Autodesk Inventor part; units mm, degrees
(part 2 of 2)
sketch "Эскиз23" plane through (0, -2, 0) normal (0, -1, 0) x (1, 0, 0)
  line L0 (-21, -26.125) -> (-21, -6.125) projected
  line L1 (-21, -16.125) -> (-28.5, -16.125) construction
  line L2 (-28.5, -13.725) -> (-33, -13.725)
  line L3 (-33, -13.725) -> (-33, -18.525)
  line L4 (-33, -18.525) -> (-28.5, -18.525)
  line L5 (-28.5, -18.525) -> (-28.5, -13.725)
  line L6 (-21, -16.125) -> (-28.5, -18.525) construction
  line L7 (-28.5, -13.725) -> (-21, -16.125) construction
  point P0 (0, 0)
  dimension "d124" = 7.5
  dimension "d125" = 4.8
  dimension "d130" = 4.5
  constraints: 14 end point, 2 horizontal, 2 midpoint, 2 parallel, 1 equal length, 1 perpendicular
  measures "d124" distance of L1.start L1.end
  measures "d125" distance between parallel lines of L2 L4
  measures "d130" distance between parallel lines of L3 L5
sketch "Эскиз25" plane through (-56.2, -2, -32.25) normal (-1, 0, 0) x (0, 0, 1)
  line L0 (2.125, 0) -> (30.125, 0) construction
  line L1 (30.125, 0) -> (30.125, 47.7) construction
  line L2 (30.125, 47.7) -> (2.125, 47.7) construction
  line L3 (2.125, 47.7) -> (2.125, 0) construction
  line L4 (26.125, 43.7) -> (26.125, 4) construction
  line L5 (26.125, 4) -> (6.125, 4) construction
  line L6 (6.125, 4) -> (6.125, 43.7) construction
  line L7 (6.125, 43.7) -> (26.125, 43.7) construction
  line L8 (30.125, 47.7) -> (31.625, 49.2) construction
  line L9 (30.125, 47.7) -> (26.125, 43.7) construction
  line L10 (26.125, 4) -> (26.125, 43.7) construction
  line L11 (26.125, 4) -> (6.125, 43.7) construction
  line L12 (26.125, 43.7) -> (6.125, 4) construction
  line L13 (16.125, 23.85) -> (26.125, 23.85) construction
  line L14 (16.125, 23.85) -> (16.125, 43.7) construction
  line L15 (6.125, 43.7) -> (26.125, 43.7) construction
  circle A0 centre (27.7819, 45.3569) radius 2.3431 construction
  circle A1 centre (27.7819, 45.3569) radius 1.05
  circle A2 centre (4.4681, 45.3569) radius 1.05
  circle A3 centre (27.7819, 2.3431) radius 1.05
  circle A4 centre (4.4681, 2.3431) radius 1.05
  point P0 (32.25, 2)
  dimension "d131" = 2.1
  constraints: 10 end point, 4 centre point, 3 midpoint, 3 symmetric about line, 1 coincident, 1 collinear, 1 horizontal, 1 point on line, 6 other
  measures "d131" diameter of A1
sketch "Эскиз26" plane through (-46.2, -2, -32.25) normal (-1, 0, 0) x (0, 0, 1)
  circle A0 centre (21.0926, -11.2426) radius 1.05
  line L0 (2.125, 47.7) -> (30.125, 47.7) projected
  circle A1 centre (4.4681, 45.3569) radius 1.05 projected
  line L1 (6.1624, 47.0511) -> (6.7825, 44.7367)
  line L2 (6.7825, 44.7367) -> (5.0883, 43.0425)
  line L3 (5.0883, 43.0425) -> (2.7739, 43.6626)
  line L4 (2.7739, 43.6626) -> (2.1538, 45.977)
  line L5 (2.1538, 45.977) -> (3.848, 47.6712)
  line L6 (3.848, 47.6712) -> (6.1624, 47.0511)
  line L7 (26.125, 43.7) -> (6.125, 43.7) projected
  line L8 (6.7825, 44.7367) -> (9.7458, 47.7)
  line L9 (9.7458, 47.7) -> (6.8113, 50.6345)
  line L10 (6.8113, 50.6345) -> (3.848, 47.6712)
  circle A2 centre (4.4681, 2.3431) radius 1.05 projected
  circle A3 centre (4.4681, 45.3569) radius 1.05 projected
  circle A4 centre (27.7819, 45.3569) radius 1.05 projected
  circle A5 centre (27.7819, 2.3431) radius 1.05 projected
  line L11 (2.125, 0) -> (30.125, 0) projected
  line L12 (30.125, 0) -> (30.125, 47.7) projected
  line L13 (30.125, 47.7) -> (2.125, 47.7) projected
  line L14 (2.125, 47.7) -> (2.125, 0) projected
  line L15 (26.125, 43.7) -> (26.125, 4) projected
  line L16 (26.125, 4) -> (6.125, 4) projected
  line L17 (6.125, 4) -> (6.125, 43.7) projected
  line L18 (6.125, 43.7) -> (26.125, 43.7) projected
  line L19 (30.125, 47.7) -> (30.125, 0) projected
  line L20 (0.625, 0) -> (2.125, 0) projected
  line L21 (30.125, 47.7) -> (2.125, 0) construction
  line L22 (16.125, 23.85) -> (23.6976, 23.85) construction
  line L23 (16.125, 23.85) -> (16.125, 29.0933) construction
  circle A6 centre (27.7819, 45.3569) radius 1.05
  line L24 (26.0876, 47.0511) -> (25.4675, 44.7367)
  line L25 (25.4675, 44.7367) -> (27.1617, 43.0425)
  line L26 (27.1617, 43.0425) -> (29.4761, 43.6626)
  line L27 (29.4761, 43.6626) -> (30.0962, 45.977)
  line L28 (30.0962, 45.977) -> (28.402, 47.6712)
  line L29 (28.402, 47.6712) -> (26.0876, 47.0511)
  line L30 (25.4675, 44.7367) -> (22.5042, 47.7)
  line L31 (22.5042, 47.7) -> (25.4387, 50.6345)
  line L32 (25.4387, 50.6345) -> (28.402, 47.6712)
  circle A7 centre (27.7819, 45.3569) radius 1.05
  line L33 (2.125, 0) -> (30.125, 0)
  circle A8 centre (4.4681, 2.3431) radius 1.05
  line L34 (6.1624, 0.6489) -> (6.7825, 2.9633)
  line L35 (6.7825, 2.9633) -> (5.0883, 4.6575)
  line L36 (5.0883, 4.6575) -> (2.7739, 4.0374)
  line L37 (2.7739, 4.0374) -> (2.1538, 1.723)
  line L38 (2.1538, 1.723) -> (3.848, 0.0288)
  line L39 (3.848, 0.0288) -> (6.1624, 0.6489)
  line L40 (26.125, 4) -> (6.125, 4)
  line L41 (6.7825, 2.9633) -> (9.7458, 0)
  line L42 (9.7458, 0) -> (6.8113, -2.9345)
  line L43 (6.8113, -2.9345) -> (3.848, 0.0288)
  circle A9 centre (4.4681, 2.3431) radius 1.05
  circle A10 centre (27.7819, 2.3431) radius 1.05
  line L44 (30.125, 0) -> (2.125, 0)
  line L45 (6.125, 4) -> (26.125, 4)
  circle A11 centre (27.7819, 2.3431) radius 1.05
  circle A12 centre (27.7819, 2.3431) radius 1.05
  line L46 (25.4675, 2.9633) -> (27.1617, 4.6575)
  line L47 (25.4675, 2.9633) -> (22.5042, 0)
  line L48 (27.1617, 4.6575) -> (29.4761, 4.0374)
  line L49 (29.4761, 4.0374) -> (30.0962, 1.723)
  line L50 (30.0962, 1.723) -> (28.402, 0.0288)
  line L51 (26.0876, 0.6489) -> (25.4675, 2.9633)
  line L52 (22.5042, 0) -> (25.4387, -2.9345)
  line L53 (25.4387, -2.9345) -> (28.402, 0.0288)
  line L54 (28.402, 0.0288) -> (26.0876, 0.6489)
  point P0 (30.125, 47.7)
  point P1 (30.125, 47.7)
  point P2 (30.125, 0)
  point P3 (30.125, 0)
  dimension "d143" = 4.15
  dimension "d144" = 45
  constraints: 46 end point, 13 centre point, 11 coincident, 11 parallel, 10 tangent, 6 horizontal, 5 perpendicular, 1 vertical, 2 other
  measures "d143" distance between parallel lines of L2 L5
  measures "d144" angle of L2 L7
